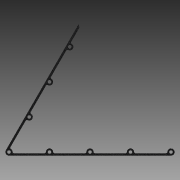
# Autodesk Inventor part: g16-strut1
Saved by Autodesk Inventor 2013 (Build 170138000, 138)
## iProperties
Created: 2013-03-23
Part Number: g16-strut1
Material: Acrylic
Document SubType Name: Modeling
Designer: Beth Scott
Density: 1 g/cm^3
d0: 1.000 ul
d2: 3.000 mm
Strut_Thickness: 2.000 mm
d12: 2.000 mm
d13: 2.000 mm
d14: 2.000 mm
Strut_MateAngle: 135.00 deg
d16: 2.000 mm
d17: 2.000 mm
Strut_Separation: 0.001 mm
d26: 2.000 mm
d27: 2.000 mm
d28: 2.000 mm
ThickLayerThickness: 6.000 mm
d30: 0.00 deg
d1: 1.000 ul
d6: 2.750 mm
d7: 0.00 deg
d8: 3.000 mm
d18: 1.000 ul
d20: 1.000 ul
d22: 0.00 deg
Bolt_HeadDiameter: 6.000 mm
LayerThickness: 2.750 mm
d4: 0.00 deg
Bolt_HoleDiameter: 3.000 mm
d19: 0.00 deg
Bolt_HeadDiameter_1: 6.000 mm
LayerThickness_1: 2.750 mm
Bolt_HoleDiameter_1: 3.000 mm
Pixel_BorderWidth_1: 1.000 mm
Pixel_Stride_1: 33.333 mm
Base_SideWidth: 133.332 mm
Pixel_BorderWidth_2: 1.000 mm
Pixel_Stride_2: 33.333 mm
d24_1: 6.000 mm
CardboardThickness: 1.750 mm
LED_StripWidth: 10.250 mm
LED_Package: 5.000 mm
LED_CapW: 2.500 mm
LED_CapH: 6.000 mm
d32: 16.667 mm
d33: 10.250 mm
LED_SlotWidth: 2.000 mm
d36: 2.000 mm
AlignmentNotchDiameter: 2.000 mm
d52: 2.000 mm
d53: 2.000 mm
LED_CapDist: 8.000 mm
d56: 16.667 mm
d61: 16.667 mm
d62: 28.867 mm
Cardboard_BorderThickness: 2.000 mm
Author: Beth Scott
Autodesk Inventor part; units mm, degrees
(part 1 of 2)
ref_plane "YZ Plane" through (0, 0, 0) normal (1, 0, 0) x (0, 1, 0)
ref_plane "XZ Plane" through (0, 0, 0) normal (0, 1, 0) x (-1, 0, 0)
ref_plane "XY Plane" through (0, 0, 0) normal (0, 0, 1) x (1, 0, 0)
sketch "Triangle Hole Template" plane through (0, 0, 0) normal (0, 0, 1) x (1, 0, 0)
  line L0 (-99.9974, -57.7156) -> (-66.6644, -57.7156) construction
  line L1 (-66.6644, -57.7156) -> (-83.3309, -86.5829) construction
  line L2 (-83.3309, -86.5829) -> (-99.9974, -57.7156) construction
  line L3 (-99.1314, -58.2156) -> (-67.5304, -58.2156) construction
  line L4 (-67.5304, -58.2156) -> (-83.3309, -85.5829) construction
  line L5 (-83.3309, -85.5829) -> (-99.1314, -58.2156) construction
  line L6 (-83.3309, -58.2156) -> (-83.3309, -57.7156) construction
  line L7 (-75.4307, -71.8992) -> (-74.9976, -72.1492) construction
  line L8 (-91.2311, -71.8992) -> (-91.6641, -72.1492) construction
  arc A0 (-68.5696, -60.0156) -> (-69.6089, -58.2156) centre (-69.6089, -59.4156) ccw
  arc A1 (-84.3701, -83.7829) -> (-82.2917, -83.7829) centre (-83.3309, -83.1829) ccw
  arc A2 (-97.0529, -58.2156) -> (-98.0921, -60.0156) centre (-97.0529, -59.4156) ccw
  line L9 (-97.0529, -58.2156) -> (-69.6089, -58.2156)
  line L10 (-68.5696, -60.0156) -> (-82.2917, -83.7829)
  line L11 (-84.3701, -83.7829) -> (-98.0921, -60.0156)
  circle A3 centre (-98.4385, -58.6156) radius 0.4 construction
  line L12 (-98.0921, -58.8156) -> (-98.785, -58.4156) construction
  circle A4 centre (-99.9974, -57.7156) radius 3 construction
  line L13 (-83.3309, -57.7156) -> (-83.3309, -57.2156) construction
  line L14 (-98.0921, -58.8156) -> (-97.3993, -59.2156) construction
  point P0 (-85.6081, -66.0431)
sketch "LED Slot Spacer" plane through (0, 0, 0) normal (0, 0, 1) x (1, 0, 0)
  line L0 (134.5658, -38.3134) -> (132.5658, -38.3134) construction
  point P0 (133.5658, -38.3134)
  point P1 (133.5658, -38.3134)
  dimension "d36" = 2
  measures "d36" distance of L0.start L0.end
sketch "LED Slot" plane through (0, 0, 0) normal (0, 0, 1) x (1, 0, 0)
  line L0 (126.9917, -69.5033) -> (126.9917, -59.2533)
  line L1 (128.9917, -69.5033) -> (128.9917, -59.2533)
  arc A0 (126.9917, -69.5033) -> (128.9917, -69.5033) centre (127.9917, -69.5033) ccw
  arc A1 (128.9917, -59.2533) -> (126.9917, -59.2533) centre (127.9917, -59.2533) ccw
  point P0 (127.9917, -64.3783)
  dimension "d33" = 10.25
  dimension "LED_SlotWidth" = 2
  measures "d33" distance of L0.start L0.end
  measures "LED_SlotWidth" distance of L0.start L1.start
sketch "LED Keepout Regions" plane through (0, 0, 0) normal (0, 0, 1) x (1, 0, 0)
  line L0 (120.8464, -124.1742) -> (104.1799, -124.1742) construction
  line L1 (104.1799, -124.1742) -> (104.1799, -113.9242) construction
  line L2 (104.1799, -113.9242) -> (120.8464, -113.9242) construction
  line L3 (120.8464, -113.9242) -> (120.8464, -124.1742) construction
  line L4 (115.0132, -121.5492) -> (110.0132, -121.5492) construction
  line L5 (110.0132, -121.5492) -> (110.0132, -116.5492) construction
  line L6 (110.0132, -116.5492) -> (115.0132, -116.5492) construction
  line L7 (115.0132, -116.5492) -> (115.0132, -121.5492) construction
  line L8 (112.5132, -124.1742) -> (112.5132, -113.9242) construction
  line L9 (120.8464, -119.0492) -> (104.1799, -119.0492) construction
  line L10 (109.5132, -122.0492) -> (107.0132, -122.0492) construction
  line L11 (107.0132, -122.0492) -> (107.0132, -116.0492) construction
  line L12 (107.0132, -116.0492) -> (109.5132, -116.0492) construction
  line L13 (109.5132, -116.0492) -> (109.5132, -122.0492) construction
  line L14 (117.0132, -113.9242) -> (117.0132, -124.1742) construction
  line L15 (105.0132, -113.9242) -> (105.0132, -124.1742) construction
  point P0 (111.5921, -119.1808)
  point P1 (115.0132, -119.0492)
  point P2 (112.5132, -121.5492)
  point P3 (109.5132, -119.0492)
  dimension "LED_StripWidth" = 10.25
  dimension "LED_Package" = 5
  dimension "LED_CapW" = 2.5
  dimension "LED_CapH" = 6
  dimension "d32" = 16.6665
  dimension "d52" = 2
  dimension "d53" = 2
  dimension "LED_CapDist" = 8
  measures "LED_StripWidth" distance of L2.end L0.start
  measures "LED_Package" distance of L4.start L4.end
  measures "LED_CapW" distance of L10.start L10.end
  measures "LED_CapH" distance of L10.end L11.end
  measures "d32" distance of L1.end L2.end
  measures "d52" distance between parallel lines of L11 L15
  measures "d53" distance between parallel lines of L14 L7
  measures "LED_CapDist" distance between parallel lines of L7 L11
sketch "Triangle Hole Template_1" plane through (0, 0, 0) normal (0, 0, 1) x (1, 0, 0)
  line L0 (-99.9974, -57.7156) -> (-66.6644, -57.7156) construction
  line L1 (-66.6644, -57.7156) -> (-83.3309, -86.5829) construction
  line L2 (-83.3309, -86.5829) -> (-99.9974, -57.7156) construction
  line L3 (-99.1314, -58.2156) -> (-67.5304, -58.2156) construction
  line L4 (-83.3309, -57.7156) -> (-83.3309, -57.2156) construction
  line L5 (-98.0921, -58.8156) -> (-97.3993, -59.2156) construction
  line L6 (-67.5304, -58.2156) -> (-83.3309, -85.5829) construction
  line L7 (-83.3309, -85.5829) -> (-99.1314, -58.2156) construction
  line L8 (-83.3309, -58.2156) -> (-83.3309, -57.7156) construction
  line L9 (-75.4307, -71.8992) -> (-74.9976, -72.1492) construction
  line L10 (-91.2311, -71.8992) -> (-91.6641, -72.1492) construction
  arc A0 (-68.5696, -60.0156) -> (-69.6089, -58.2156) centre (-69.6089, -59.4156) ccw
  arc A1 (-84.3701, -83.7829) -> (-82.2917, -83.7829) centre (-83.3309, -83.1829) ccw
  arc A2 (-97.0529, -58.2156) -> (-98.0921, -60.0156) centre (-97.0529, -59.4156) ccw
  line L11 (-97.0529, -58.2156) -> (-69.6089, -58.2156)
  line L12 (-68.5696, -60.0156) -> (-82.2917, -83.7829)
  line L13 (-84.3701, -83.7829) -> (-98.0921, -60.0156)
  circle A3 centre (-98.4385, -58.6156) radius 0.4 construction
  line L14 (-98.0921, -58.8156) -> (-98.785, -58.4156) construction
  circle A4 centre (-99.9974, -57.7156) radius 3 construction
  point P0 (-85.6081, -66.0431)
sketch "Triangle Hole Template x16" plane through (0, 0, 0) normal (0, 0, 1) x (1, 0, 0)
  line L0 (-99.9974, -57.7156) -> (-66.6644, -57.7156) construction
  line L1 (-66.6644, -57.7156) -> (-83.3309, -86.5829) construction
  line L2 (-83.3309, -86.5829) -> (-99.9974, -57.7156) construction
  line L3 (-99.1314, -58.2156) -> (-67.5304, -58.2156) construction
  line L4 (-67.5304, -58.2156) -> (-83.3309, -85.5829) construction
  line L5 (-83.3309, -85.5829) -> (-99.1314, -58.2156) construction
  line L6 (-83.3309, -58.2156) -> (-83.3309, -57.7156) construction
  line L7 (-75.4307, -71.8992) -> (-74.9976, -72.1492) construction
  line L8 (-91.2311, -71.8992) -> (-91.6641, -72.1492) construction
  arc A0 (-68.5696, -60.0156) -> (-69.6089, -58.2156) centre (-69.6089, -59.4156) ccw
  arc A1 (-84.3701, -83.7829) -> (-82.2917, -83.7829) centre (-83.3309, -83.1829) ccw
  arc A2 (-97.0529, -58.2156) -> (-98.0921, -60.0156) centre (-97.0529, -59.4156) ccw
  line L9 (-97.0529, -58.2156) -> (-69.6089, -58.2156)
  line L10 (-68.5696, -60.0156) -> (-82.2917, -83.7829)
  line L11 (-84.3701, -83.7829) -> (-98.0921, -60.0156)
  circle A3 centre (-98.4385, -58.6156) radius 0.4 construction
  line L12 (-98.0921, -58.8156) -> (-98.785, -58.4156) construction
  circle A4 centre (-99.9974, -57.7156) radius 3 construction
  line L13 (-83.3309, -57.7156) -> (-83.3309, -57.2156) construction
  line L14 (-98.0921, -58.8156) -> (-97.3993, -59.2156) construction
  line L15 (-83.3309, -86.5829) -> (-49.9979, -86.5829) construction
  line L16 (-49.9979, -86.5829) -> (-66.6644, -115.4501) construction
  line L17 (-66.6644, -115.4501) -> (-83.3309, -86.5829) construction
  line L18 (-82.4649, -87.0829) -> (-50.8639, -87.0829) construction
  line L19 (-50.8639, -87.0829) -> (-66.6644, -114.4501) construction
  line L20 (-66.6644, -114.4501) -> (-82.4649, -87.0829) construction
  line L21 (-66.6644, -87.0829) -> (-66.6644, -86.5829) construction
  line L22 (-58.7642, -100.7665) -> (-58.3311, -101.0165) construction
  line L23 (-74.5646, -100.7665) -> (-74.9976, -101.0165) construction
  arc A5 (-51.9031, -88.8829) -> (-52.9424, -87.0829) centre (-52.9424, -88.2829) ccw
  arc A6 (-67.7036, -112.6501) -> (-65.6252, -112.6501) centre (-66.6644, -112.0501) ccw
  arc A7 (-80.3864, -87.0829) -> (-81.4256, -88.8829) centre (-80.3864, -88.2829) ccw
  line L24 (-80.3864, -87.0829) -> (-52.9424, -87.0829)
  line L25 (-51.9031, -88.8829) -> (-65.6252, -112.6501)
  line L26 (-67.7036, -112.6501) -> (-81.4256, -88.8829)
  circle A8 centre (-81.772, -87.4829) radius 0.4 construction
  line L27 (-81.4256, -87.6829) -> (-82.1185, -87.2829) construction
  circle A9 centre (-83.3309, -86.5829) radius 3 construction
  line L28 (-66.6644, -86.5829) -> (-66.6644, -86.0829) construction
  line L29 (-81.4256, -87.6829) -> (-80.7328, -88.0829) construction
  line L30 (-66.6676, -57.7533) -> (-33.3346, -57.7533) construction
  line L31 (-33.3346, -57.7533) -> (-50.0011, -86.6205) construction
  line L32 (-50.0011, -86.6205) -> (-66.6676, -57.7533) construction
  line L33 (-65.8016, -58.2533) -> (-34.2006, -58.2533) construction
  line L34 (-34.2006, -58.2533) -> (-50.0011, -85.6205) construction
  line L35 (-50.0011, -85.6205) -> (-65.8016, -58.2533) construction
  line L36 (-50.0011, -58.2533) -> (-50.0011, -57.7533) construction
  line L37 (-42.1009, -71.9369) -> (-41.6679, -72.1869) construction
  line L38 (-57.9013, -71.9369) -> (-58.3344, -72.1869) construction
  arc A10 (-35.2399, -60.0533) -> (-36.2791, -58.2533) centre (-36.2791, -59.4533) ccw
  arc A11 (-51.0403, -83.8205) -> (-48.9619, -83.8205) centre (-50.0011, -83.2205) ccw
  arc A12 (-63.7231, -58.2533) -> (-64.7624, -60.0533) centre (-63.7231, -59.4533) ccw
  line L39 (-63.7231, -58.2533) -> (-36.2791, -58.2533)
  line L40 (-35.2399, -60.0533) -> (-48.9619, -83.8205)
  line L41 (-51.0403, -83.8205) -> (-64.7624, -60.0533)
  circle A13 centre (-65.1088, -58.6533) radius 0.4 construction
  line L42 (-64.7624, -58.8533) -> (-65.4552, -58.4533) construction
  circle A14 centre (-66.6676, -57.7533) radius 3 construction
  line L43 (-50.0011, -57.7533) -> (-50.0011, -57.2533) construction
  line L44 (-64.7624, -58.8533) -> (-64.0695, -59.2533) construction
  line L45 (-50.0011, -86.6205) -> (-83.3341, -86.6205) construction
  line L46 (-83.3341, -86.6205) -> (-66.6676, -57.7533) construction
  line L47 (-66.6676, -57.7533) -> (-50.0011, -86.6205) construction
  line L48 (-50.8671, -86.1205) -> (-82.4681, -86.1205) construction
  line L49 (-82.4681, -86.1205) -> (-66.6676, -58.7533) construction
  line L50 (-66.6676, -58.7533) -> (-50.8671, -86.1205) construction
  line L51 (-66.6676, -86.1205) -> (-66.6676, -86.6205) construction
  line L52 (-74.5678, -72.4369) -> (-75.0009, -72.1869) construction
  line L53 (-58.7674, -72.4369) -> (-58.3344, -72.1869) construction
  arc A15 (-81.4289, -84.3205) -> (-80.3896, -86.1205) centre (-80.3896, -84.9205) ccw
  arc A16 (-65.6284, -60.5533) -> (-67.7068, -60.5533) centre (-66.6676, -61.1533) ccw
  arc A17 (-52.9456, -86.1205) -> (-51.9064, -84.3205) centre (-52.9456, -84.9205) ccw
  line L54 (-52.9456, -86.1205) -> (-80.3896, -86.1205)
  line L55 (-81.4289, -84.3205) -> (-67.7068, -60.5533)
  line L56 (-65.6284, -60.5533) -> (-51.9064, -84.3205)
  circle A18 centre (-51.56, -85.7205) radius 0.4 construction
  line L57 (-51.9064, -85.5205) -> (-51.2135, -85.9205) construction
  circle A19 centre (-50.0011, -86.6205) radius 3 construction
  line L58 (-66.6676, -86.6205) -> (-66.6676, -87.1205) construction
  line L59 (-51.9064, -85.5205) -> (-52.5992, -85.1205) construction
  line L60 (-33.3346, -57.7533) -> (-66.6676, -57.7533) construction
  line L61 (-66.6676, -57.7533) -> (-50.0011, -28.886) construction
  line L62 (-50.0011, -28.886) -> (-33.3346, -57.7533) construction
  line L63 (-34.2006, -57.2533) -> (-65.8016, -57.2533) construction
  line L64 (-65.8016, -57.2533) -> (-50.0011, -29.886) construction
  line L65 (-50.0011, -29.886) -> (-34.2006, -57.2533) construction
  line L66 (-50.0011, -57.2533) -> (-50.0011, -57.7533) construction
  line L67 (-57.9013, -43.5697) -> (-58.3344, -43.3197) construction
  line L68 (-42.1009, -43.5697) -> (-41.6679, -43.3197) construction
  arc A20 (-64.7624, -55.4533) -> (-63.7231, -57.2533) centre (-63.7231, -56.0533) ccw
  arc A21 (-48.9619, -31.686) -> (-51.0403, -31.686) centre (-50.0011, -32.286) ccw
  arc A22 (-36.2791, -57.2533) -> (-35.2399, -55.4533) centre (-36.2791, -56.0533) ccw
  line L69 (-36.2791, -57.2533) -> (-63.7231, -57.2533)
  line L70 (-64.7624, -55.4533) -> (-51.0403, -31.686)
  line L71 (-48.9619, -31.686) -> (-35.2399, -55.4533)
  circle A23 centre (-34.8935, -56.8533) radius 0.4 construction
  line L72 (-35.2399, -56.6533) -> (-34.547, -57.0533) construction
  circle A24 centre (-33.3346, -57.7533) radius 3 construction
  line L73 (-50.0011, -57.7533) -> (-50.0011, -58.2533) construction
  line L74 (-35.2399, -56.6533) -> (-35.9327, -56.2533) construction
  line L75 (-66.6676, -57.7156) -> (-100.0006, -57.7156) construction
  line L76 (-100.0006, -57.7156) -> (-83.3341, -28.8484) construction
  line L77 (-83.3341, -28.8484) -> (-66.6676, -57.7156) construction
  line L78 (-67.5336, -57.2156) -> (-99.1346, -57.2156) construction
  line L79 (-99.1346, -57.2156) -> (-83.3341, -29.8484) construction
  line L80 (-83.3341, -29.8484) -> (-67.5336, -57.2156) construction
  line L81 (-83.3341, -57.2156) -> (-83.3341, -57.7156) construction
  line L82 (-91.2343, -43.532) -> (-91.6674, -43.282) construction
  line L83 (-75.4339, -43.532) -> (-75.0009, -43.282) construction
  arc A25 (-98.0954, -55.4156) -> (-97.0561, -57.2156) centre (-97.0561, -56.0156) ccw
  arc A26 (-82.2949, -31.6484) -> (-84.3733, -31.6484) centre (-83.3341, -32.2484) ccw
  arc A27 (-69.6121, -57.2156) -> (-68.5729, -55.4156) centre (-69.6121, -56.0156) ccw
  line L84 (-69.6121, -57.2156) -> (-97.0561, -57.2156)
  line L85 (-98.0954, -55.4156) -> (-84.3733, -31.6484)
  line L86 (-82.2949, -31.6484) -> (-68.5729, -55.4156)
  circle A28 centre (-68.2265, -56.8156) radius 0.4 construction
  line L87 (-68.5729, -56.6156) -> (-67.88, -57.0156) construction
  circle A29 centre (-66.6676, -57.7156) radius 3 construction
  line L88 (-83.3341, -57.7156) -> (-83.3341, -58.2156) construction
  line L89 (-68.5729, -56.6156) -> (-69.2657, -56.2156) construction
  line L90 (-83.3186, -28.8752) -> (-116.6516, -28.8752) construction
  line L91 (-116.6516, -28.8752) -> (-99.9851, -0.008) construction
  line L92 (-99.9851, -0.008) -> (-83.3186, -28.8752) construction
  line L93 (-84.1846, -28.3752) -> (-115.7856, -28.3752) construction
  line L94 (-115.7856, -28.3752) -> (-99.9851, -1.008) construction
  line L95 (-99.9851, -1.008) -> (-84.1846, -28.3752) construction
  line L96 (-99.9851, -28.3752) -> (-99.9851, -28.8752) construction
  line L97 (-107.8853, -14.6916) -> (-108.3184, -14.4416) construction
  line L98 (-92.0849, -14.6916) -> (-91.6519, -14.4416) construction
  arc A30 (-114.7464, -26.5752) -> (-113.7071, -28.3752) centre (-113.7071, -27.1752) ccw
  arc A31 (-98.9459, -2.808) -> (-101.0243, -2.808) centre (-99.9851, -3.408) ccw
  arc A32 (-86.2631, -28.3752) -> (-85.2239, -26.5752) centre (-86.2631, -27.1752) ccw
  line L99 (-86.2631, -28.3752) -> (-113.7071, -28.3752)
  line L100 (-114.7464, -26.5752) -> (-101.0243, -2.808)
  line L101 (-98.9459, -2.808) -> (-85.2239, -26.5752)
  circle A33 centre (-84.8775, -27.9752) radius 0.4 construction
  line L102 (-85.2239, -27.7752) -> (-84.531, -28.1752) construction
  circle A34 centre (-83.3186, -28.8752) radius 3 construction
  line L103 (-99.9851, -28.8752) -> (-99.9851, -29.3752) construction
  line L104 (-85.2239, -27.7752) -> (-85.9167, -27.3752) construction
  line L105 (-50.0011, -28.8484) -> (-83.3341, -28.8484) construction
  line L106 (-83.3341, -28.8484) -> (-66.6676, 0.0188) construction
  line L107 (-66.6676, 0.0188) -> (-50.0011, -28.8484) construction
  line L108 (-50.8671, -28.3484) -> (-82.4681, -28.3484) construction
  line L109 (-82.4681, -28.3484) -> (-66.6676, -0.9812) construction
  line L110 (-66.6676, -0.9812) -> (-50.8671, -28.3484) construction
  line L111 (-66.6676, -28.3484) -> (-66.6676, -28.8484) construction
  line L112 (-74.5678, -14.6648) -> (-75.0009, -14.4148) construction
  line L113 (-58.7674, -14.6648) -> (-58.3344, -14.4148) construction
  arc A35 (-81.4289, -26.5484) -> (-80.3896, -28.3484) centre (-80.3896, -27.1484) ccw
  arc A36 (-65.6284, -2.7812) -> (-67.7068, -2.7812) centre (-66.6676, -3.3812) ccw
  arc A37 (-52.9456, -28.3484) -> (-51.9064, -26.5484) centre (-52.9456, -27.1484) ccw
  line L114 (-52.9456, -28.3484) -> (-80.3896, -28.3484)
  line L115 (-81.4289, -26.5484) -> (-67.7068, -2.7812)
  line L116 (-65.6284, -2.7812) -> (-51.9064, -26.5484)
  circle A38 centre (-51.56, -27.9484) radius 0.4 construction
  line L117 (-51.9064, -27.7484) -> (-51.2135, -28.1484) construction
  circle A39 centre (-50.0011, -28.8484) radius 3 construction
  line L118 (-66.6676, -28.8484) -> (-66.6676, -29.3484) construction
  line L119 (-51.9064, -27.7484) -> (-52.5992, -27.3484) construction
  line L120 (-16.6681, -28.8484) -> (-50.0011, -28.8484) construction
  line L121 (-50.0011, -28.8484) -> (-33.3346, 0.0188) construction
  line L122 (-33.3346, 0.0188) -> (-16.6681, -28.8484) construction
  line L123 (-17.5341, -28.3484) -> (-49.1351, -28.3484) construction
  line L124 (-49.1351, -28.3484) -> (-33.3346, -0.9812) construction
  line L125 (-33.3346, -0.9812) -> (-17.5341, -28.3484) construction
  line L126 (-33.3346, -28.3484) -> (-33.3346, -28.8484) construction
  line L127 (-41.2348, -14.6648) -> (-41.6679, -14.4148) construction
  line L128 (-25.4344, -14.6648) -> (-25.0014, -14.4148) construction
  arc A40 (-48.0959, -26.5484) -> (-47.0566, -28.3484) centre (-47.0566, -27.1484) ccw
  arc A41 (-32.2954, -2.7812) -> (-34.3738, -2.7812) centre (-33.3346, -3.3812) ccw
  arc A42 (-19.6126, -28.3484) -> (-18.5734, -26.5484) centre (-19.6126, -27.1484) ccw
  line L129 (-19.6126, -28.3484) -> (-47.0566, -28.3484)
  line L130 (-48.0959, -26.5484) -> (-34.3738, -2.7812)
  line L131 (-32.2954, -2.7812) -> (-18.5734, -26.5484)
  circle A43 centre (-18.227, -27.9484) radius 0.4 construction
  line L132 (-18.5734, -27.7484) -> (-17.8805, -28.1484) construction
  circle A44 centre (-16.6681, -28.8484) radius 3 construction
  line L133 (-33.3346, -28.8484) -> (-33.3346, -29.3484) construction
  line L134 (-18.5734, -27.7484) -> (-19.2662, -27.3484) construction
  line L135 (-49.9979, -28.8484) -> (-16.6649, -28.8484) construction
  line L136 (-16.6649, -28.8484) -> (-33.3314, -57.7156) construction
  line L137 (-33.3314, -57.7156) -> (-49.9979, -28.8484) construction
  line L138 (-49.1319, -29.3484) -> (-17.5309, -29.3484) construction
  line L139 (-17.5309, -29.3484) -> (-33.3314, -56.7156) construction
  line L140 (-33.3314, -56.7156) -> (-49.1319, -29.3484) construction
  line L141 (-33.3314, -29.3484) -> (-33.3314, -28.8484) construction
  line L142 (-25.4312, -43.032) -> (-24.9981, -43.282) construction
  line L143 (-41.2316, -43.032) -> (-41.6646, -43.282) construction
  arc A45 (-18.5701, -31.1484) -> (-19.6094, -29.3484) centre (-19.6094, -30.5484) ccw
  arc A46 (-34.3706, -54.9156) -> (-32.2922, -54.9156) centre (-33.3314, -54.3156) ccw
  arc A47 (-47.0534, -29.3484) -> (-48.0926, -31.1484) centre (-47.0534, -30.5484) ccw
  line L144 (-47.0534, -29.3484) -> (-19.6094, -29.3484)
  line L145 (-18.5701, -31.1484) -> (-32.2922, -54.9156)
  line L146 (-34.3706, -54.9156) -> (-48.0926, -31.1484)
  circle A48 centre (-48.439, -29.7484) radius 0.4 construction
  line L147 (-48.0926, -29.9484) -> (-48.7855, -29.5484) construction
  circle A49 centre (-49.9979, -28.8484) radius 3 construction
  line L148 (-33.3314, -28.8484) -> (-33.3314, -28.3484) construction
  line L149 (-48.0926, -29.9484) -> (-47.3998, -30.3484) construction
  line L150 (-66.6676, 0.0188) -> (-33.3346, 0.0188) construction
  line L151 (-33.3346, 0.0188) -> (-50.0011, -28.8484) construction
  line L152 (-50.0011, -28.8484) -> (-66.6676, 0.0188) construction
  line L153 (-65.8016, -0.4812) -> (-34.2006, -0.4812) construction
  line L154 (-34.2006, -0.4812) -> (-50.0011, -27.8484) construction
  line L155 (-50.0011, -27.8484) -> (-65.8016, -0.4812) construction
  line L156 (-50.0011, -0.4812) -> (-50.0011, 0.0188) construction
  line L157 (-42.1009, -14.1648) -> (-41.6679, -14.4148) construction
  line L158 (-57.9013, -14.1648) -> (-58.3344, -14.4148) construction
  arc A50 (-35.2399, -2.2812) -> (-36.2791, -0.4812) centre (-36.2791, -1.6812) ccw
  arc A51 (-51.0403, -26.0484) -> (-48.9619, -26.0484) centre (-50.0011, -25.4484) ccw
  arc A52 (-63.7231, -0.4812) -> (-64.7624, -2.2812) centre (-63.7231, -1.6812) ccw
  line L159 (-63.7231, -0.4812) -> (-36.2791, -0.4812)
  line L160 (-35.2399, -2.2812) -> (-48.9619, -26.0484)
  line L161 (-51.0403, -26.0484) -> (-64.7624, -2.2812)
  circle A53 centre (-65.1088, -0.8812) radius 0.4 construction
  line L162 (-64.7624, -1.0812) -> (-65.4552, -0.6812) construction
  circle A54 centre (-66.6676, 0.0188) radius 3 construction
  line L163 (-50.0011, 0.0188) -> (-50.0011, 0.5188) construction
  line L164 (-64.7624, -1.0812) -> (-64.0695, -1.4812) construction
  line L165 (-33.3314, 0.0188) -> (0.0016, 0.0188) construction
  line L166 (0.0016, 0.0188) -> (-16.6649, -28.8484) construction
  line L167 (-16.6649, -28.8484) -> (-33.3314, 0.0188) construction
  line L168 (-32.4654, -0.4812) -> (-0.8644, -0.4812) construction
  line L169 (-0.8644, -0.4812) -> (-16.6649, -27.8484) construction
  line L170 (-16.6649, -27.8484) -> (-32.4654, -0.4812) construction
  line L171 (-16.6649, -0.4812) -> (-16.6649, 0.0188) construction
  line L172 (-8.7647, -14.1648) -> (-8.3316, -14.4148) construction
  line L173 (-24.5651, -14.1648) -> (-24.9981, -14.4148) construction
  arc A55 (-1.9036, -2.2812) -> (-2.9429, -0.4812) centre (-2.9429, -1.6812) ccw
  arc A56 (-17.7041, -26.0484) -> (-15.6257, -26.0484) centre (-16.6649, -25.4484) ccw
  arc A57 (-30.3869, -0.4812) -> (-31.4261, -2.2812) centre (-30.3869, -1.6812) ccw
  line L174 (-30.3869, -0.4812) -> (-2.9429, -0.4812)
  line L175 (-1.9036, -2.2812) -> (-15.6257, -26.0484)
  line L176 (-17.7041, -26.0484) -> (-31.4261, -2.2812)
  circle A58 centre (-31.7725, -0.8812) radius 0.4 construction
  line L177 (-31.4261, -1.0812) -> (-32.119, -0.6812) construction
  circle A59 centre (-33.3314, 0.0188) radius 3 construction
  line L178 (-16.6649, 0.0188) -> (-16.6649, 0.5188) construction
  line L179 (-31.4261, -1.0812) -> (-30.7333, -1.4812) construction
  line L180 (-83.317, -28.8188) -> (-49.984, -28.8188) construction
  line L181 (-49.984, -28.8188) -> (-66.6505, -57.686) construction
  line L182 (-66.6505, -57.686) -> (-83.317, -28.8188) construction
  line L183 (-82.451, -29.3188) -> (-50.85, -29.3188) construction
  line L184 (-50.85, -29.3188) -> (-66.6505, -56.686) construction
  line L185 (-66.6505, -56.686) -> (-82.451, -29.3188) construction
  line L186 (-66.6505, -29.3188) -> (-66.6505, -28.8188) construction
  line L187 (-58.7503, -43.0024) -> (-58.3173, -43.2524) construction
  line L188 (-74.5507, -43.0024) -> (-74.9838, -43.2524) construction
  arc A60 (-51.8893, -31.1188) -> (-52.9285, -29.3188) centre (-52.9285, -30.5188) ccw
  arc A61 (-67.6897, -54.886) -> (-65.6113, -54.886) centre (-66.6505, -54.286) ccw
  arc A62 (-80.3725, -29.3188) -> (-81.4117, -31.1188) centre (-80.3725, -30.5188) ccw
  line L189 (-80.3725, -29.3188) -> (-52.9285, -29.3188)
  line L190 (-51.8893, -31.1188) -> (-65.6113, -54.886)
  line L191 (-67.6897, -54.886) -> (-81.4117, -31.1188)
  circle A63 centre (-81.7582, -29.7188) radius 0.4 construction
  line L192 (-81.4117, -29.9188) -> (-82.1046, -29.5188) construction
  circle A64 centre (-83.317, -28.8188) radius 3 construction
  line L193 (-66.6505, -28.8188) -> (-66.6505, -28.3188) construction
  line L194 (-81.4117, -29.9188) -> (-80.7189, -30.3188) construction
  line L195 (-99.9974, 0.0188) -> (-66.6644, 0.0188) construction
  line L196 (-66.6644, 0.0188) -> (-83.3309, -28.8484) construction
  line L197 (-83.3309, -28.8484) -> (-99.9974, 0.0188) construction
  line L198 (-99.1314, -0.4812) -> (-67.5304, -0.4812) construction
  line L199 (-67.5304, -0.4812) -> (-83.3309, -27.8484) construction
  line L200 (-83.3309, -27.8484) -> (-99.1314, -0.4812) construction
  line L201 (-83.3309, -0.4812) -> (-83.3309, 0.0188) construction
  line L202 (-75.4307, -14.1648) -> (-74.9976, -14.4148) construction
  line L203 (-91.2311, -14.1648) -> (-91.6641, -14.4148) construction
  arc A65 (-68.5696, -2.2812) -> (-69.6089, -0.4812) centre (-69.6089, -1.6812) ccw
  arc A66 (-84.3701, -26.0484) -> (-82.2917, -26.0484) centre (-83.3309, -25.4484) ccw
  arc A67 (-97.0529, -0.4812) -> (-98.0921, -2.2812) centre (-97.0529, -1.6812) ccw
  line L204 (-97.0529, -0.4812) -> (-69.6089, -0.4812)
  line L205 (-68.5696, -2.2812) -> (-82.2917, -26.0484)
  line L206 (-84.3701, -26.0484) -> (-98.0921, -2.2812)
  circle A68 centre (-98.4385, -0.8812) radius 0.4 construction
  line L207 (-98.0921, -1.0812) -> (-98.785, -0.6812) construction
  circle A69 centre (-99.9974, 0.0188) radius 3 construction
  line L208 (-83.3309, 0.0188) -> (-83.3309, 0.5188) construction
  line L209 (-98.0921, -1.0812) -> (-97.3993, -1.4812) construction
  line L210 (-133.3304, -0.008) -> (-99.9974, -0.008) construction
  line L211 (-99.9974, -0.008) -> (-116.6639, -28.8752) construction
  line L212 (-116.6639, -28.8752) -> (-133.3304, -0.008) construction
  line L213 (-132.4644, -0.508) -> (-100.8634, -0.508) construction
  line L214 (-100.8634, -0.508) -> (-116.6639, -27.8752) construction
  line L215 (-116.6639, -27.8752) -> (-132.4644, -0.508) construction
  line L216 (-116.6639, -0.508) -> (-116.6639, -0.008) construction
  line L217 (-108.7637, -14.1916) -> (-108.3306, -14.4416) construction
  line L218 (-124.5641, -14.1916) -> (-124.9971, -14.4416) construction
  arc A70 (-101.9026, -2.308) -> (-102.9419, -0.508) centre (-102.9419, -1.708) ccw
  arc A71 (-117.7031, -26.0752) -> (-115.6247, -26.0752) centre (-116.6639, -25.4752) ccw
  arc A72 (-130.3859, -0.508) -> (-131.4251, -2.308) centre (-130.3859, -1.708) ccw
  line L219 (-130.3859, -0.508) -> (-102.9419, -0.508)
  line L220 (-101.9026, -2.308) -> (-115.6247, -26.0752)
  line L221 (-117.7031, -26.0752) -> (-131.4251, -2.308)
  circle A73 centre (-131.7715, -0.908) radius 0.4 construction
  line L222 (-131.4251, -1.108) -> (-132.118, -0.708) construction
  circle A74 centre (-133.3304, -0.008) radius 3 construction
  line L223 (-116.6639, -0.008) -> (-116.6639, 0.492) construction
  line L224 (-131.4251, -1.108) -> (-130.7323, -1.508) construction
  line L225 (-116.6671, -28.8484) -> (-83.3341, -28.8484) construction
  line L226 (-83.3341, -28.8484) -> (-100.0006, -57.7156) construction
  line L227 (-100.0006, -57.7156) -> (-116.6671, -28.8484) construction
  line L228 (-115.8011, -29.3484) -> (-84.2001, -29.3484) construction
  line L229 (-84.2001, -29.3484) -> (-100.0006, -56.7156) construction
  line L230 (-100.0006, -56.7156) -> (-115.8011, -29.3484) construction
  line L231 (-100.0006, -29.3484) -> (-100.0006, -28.8484) construction
  line L232 (-92.1004, -43.032) -> (-91.6674, -43.282) construction
  line L233 (-107.9008, -43.032) -> (-108.3339, -43.282) construction
  arc A75 (-85.2394, -31.1484) -> (-86.2786, -29.3484) centre (-86.2786, -30.5484) ccw
  arc A76 (-101.0398, -54.9156) -> (-98.9614, -54.9156) centre (-100.0006, -54.3156) ccw
  arc A77 (-113.7226, -29.3484) -> (-114.7619, -31.1484) centre (-113.7226, -30.5484) ccw
  line L234 (-113.7226, -29.3484) -> (-86.2786, -29.3484)
  line L235 (-85.2394, -31.1484) -> (-98.9614, -54.9156)
  line L236 (-101.0398, -54.9156) -> (-114.7619, -31.1484)
  circle A78 centre (-115.1083, -29.7484) radius 0.4 construction
  line L237 (-114.7619, -29.9484) -> (-115.4547, -29.5484) construction
  circle A79 centre (-116.6671, -28.8484) radius 3 construction
  line L238 (-100.0006, -28.8484) -> (-100.0006, -28.3484) construction
  line L239 (-114.7619, -29.9484) -> (-114.069, -30.3484) construction
  point P0 (-67.2349, -38.1612)
sketch "LED Keepout x16" plane through (0, 0, 0) normal (0, 0, 1) x (1, 0, 0)
  line L0 (133.3347, -3) -> (0.0027, -3) construction
  line L1 (116.6682, -31.8672) -> (16.6692, -31.8672) construction
  line L2 (83.3352, -89.6017) -> (50.0022, -89.6017) construction
  line L3 (116.6682, -31.8672) -> (116.6682, -3) construction
  line L4 (100.0017, -60.7344) -> (33.3357, -60.7344) construction
  line L5 (100.0017, -60.7344) -> (100.0017, -31.8672) construction
  line L6 (83.3352, -89.6017) -> (83.3352, -60.7344) construction
  line L7 (66.6687, -118.4689) -> (66.6687, -89.6017) construction
  line L8 (50.0022, -89.6017) -> (50.0022, -3) construction
  line L9 (16.6692, -31.8672) -> (16.6692, -3) construction
  line L10 (33.3357, -60.7344) -> (33.3357, -3) construction
  line L11 (66.6687, -89.6017) -> (66.6687, -3) construction
  line L12 (83.3352, -60.7344) -> (83.3352, -3) construction
  line L13 (100.0017, -31.8672) -> (100.0017, -3) construction
  line L14 (125.0015, -22.5586) -> (108.335, -22.5586) construction
  line L15 (108.335, -22.5586) -> (108.335, -12.3086) construction
  line L16 (108.335, -12.3086) -> (125.0015, -12.3086) construction
  line L17 (125.0015, -12.3086) -> (125.0015, -22.5586) construction
  line L18 (119.1682, -19.9336) -> (114.1682, -19.9336) construction
  line L19 (114.1682, -19.9336) -> (114.1682, -14.9336) construction
  line L20 (114.1682, -14.9336) -> (119.1682, -14.9336) construction
  line L21 (119.1682, -14.9336) -> (119.1682, -19.9336) construction
  line L22 (116.6682, -22.5586) -> (116.6682, -12.3086) construction
  line L23 (125.0015, -17.4336) -> (108.335, -17.4336) construction
  line L24 (113.6682, -20.4336) -> (111.1682, -20.4336) construction
  line L25 (111.1682, -20.4336) -> (111.1682, -14.4336) construction
  line L26 (111.1682, -14.4336) -> (113.6682, -14.4336) construction
  line L27 (113.6682, -14.4336) -> (113.6682, -20.4336) construction
  line L28 (121.1682, -12.3086) -> (121.1682, -22.5586) construction
  line L29 (109.1682, -12.3086) -> (109.1682, -22.5586) construction
  line L30 (108.335, -22.5586) -> (91.6685, -22.5586) construction
  line L31 (91.6685, -22.5586) -> (91.6685, -12.3086) construction
  line L32 (91.6685, -12.3086) -> (108.335, -12.3086) construction
  line L33 (108.335, -12.3086) -> (108.335, -22.5586) construction
  line L34 (102.5017, -19.9336) -> (97.5017, -19.9336) construction
  line L35 (97.5017, -19.9336) -> (97.5017, -14.9336) construction
  line L36 (97.5017, -14.9336) -> (102.5017, -14.9336) construction
  line L37 (102.5017, -14.9336) -> (102.5017, -19.9336) construction
  line L38 (100.0017, -22.5586) -> (100.0017, -12.3086) construction
  line L39 (108.335, -17.4336) -> (91.6685, -17.4336) construction
  line L40 (97.0017, -20.4336) -> (94.5017, -20.4336) construction
  line L41 (94.5017, -20.4336) -> (94.5017, -14.4336) construction
  line L42 (94.5017, -14.4336) -> (97.0017, -14.4336) construction
  line L43 (97.0017, -14.4336) -> (97.0017, -20.4336) construction
  line L44 (104.5017, -12.3086) -> (104.5017, -22.5586) construction
  line L45 (92.5017, -12.3086) -> (92.5017, -22.5586) construction
  line L46 (91.6685, -22.5586) -> (75.002, -22.5586) construction
  line L47 (75.002, -22.5586) -> (75.002, -12.3086) construction
  line L48 (75.002, -12.3086) -> (91.6685, -12.3086) construction
  line L49 (91.6685, -12.3086) -> (91.6685, -22.5586) construction
  line L50 (85.8352, -19.9336) -> (80.8352, -19.9336) construction
  line L51 (80.8352, -19.9336) -> (80.8352, -14.9336) construction
  line L52 (80.8352, -14.9336) -> (85.8352, -14.9336) construction
  line L53 (85.8352, -14.9336) -> (85.8352, -19.9336) construction
  line L54 (83.3352, -22.5586) -> (83.3352, -12.3086) construction
  line L55 (91.6685, -17.4336) -> (75.002, -17.4336) construction
  line L56 (80.3352, -20.4336) -> (77.8352, -20.4336) construction
  line L57 (77.8352, -20.4336) -> (77.8352, -14.4336) construction
  line L58 (77.8352, -14.4336) -> (80.3352, -14.4336) construction
  line L59 (80.3352, -14.4336) -> (80.3352, -20.4336) construction
  line L60 (87.8352, -12.3086) -> (87.8352, -22.5586) construction
  line L61 (75.8352, -12.3086) -> (75.8352, -22.5586) construction
  line L62 (75.002, -22.5586) -> (58.3355, -22.5586) construction
  line L63 (58.3355, -22.5586) -> (58.3355, -12.3086) construction
  line L64 (58.3355, -12.3086) -> (75.002, -12.3086) construction
  line L65 (75.002, -12.3086) -> (75.002, -22.5586) construction
  line L66 (69.1687, -19.9336) -> (64.1687, -19.9336) construction
  line L67 (64.1687, -19.9336) -> (64.1687, -14.9336) construction
  line L68 (64.1687, -14.9336) -> (69.1687, -14.9336) construction
  line L69 (69.1687, -14.9336) -> (69.1687, -19.9336) construction
  line L70 (66.6687, -22.5586) -> (66.6687, -12.3086) construction
  line L71 (75.002, -17.4336) -> (58.3355, -17.4336) construction
  line L72 (63.6687, -20.4336) -> (61.1687, -20.4336) construction
  line L73 (61.1687, -20.4336) -> (61.1687, -14.4336) construction
  line L74 (61.1687, -14.4336) -> (63.6687, -14.4336) construction
  line L75 (63.6687, -14.4336) -> (63.6687, -20.4336) construction
  line L76 (71.1687, -12.3086) -> (71.1687, -22.5586) construction
  line L77 (59.1687, -12.3086) -> (59.1687, -22.5586) construction
  line L78 (41.669, -22.5586) -> (25.0025, -22.5586) construction
  line L79 (25.0025, -22.5586) -> (25.0025, -12.3086) construction
  line L80 (25.0025, -12.3086) -> (41.669, -12.3086) construction
  line L81 (41.669, -12.3086) -> (41.669, -22.5586) construction
  line L82 (35.8357, -19.9336) -> (30.8357, -19.9336) construction
  line L83 (30.8357, -19.9336) -> (30.8357, -14.9336) construction
  line L84 (30.8357, -14.9336) -> (35.8357, -14.9336) construction
  line L85 (35.8357, -14.9336) -> (35.8357, -19.9336) construction
  line L86 (33.3357, -22.5586) -> (33.3357, -12.3086) construction
  line L87 (41.669, -17.4336) -> (25.0025, -17.4336) construction
  line L88 (30.3357, -20.4336) -> (27.8357, -20.4336) construction
  line L89 (27.8357, -20.4336) -> (27.8357, -14.4336) construction
  line L90 (27.8357, -14.4336) -> (30.3357, -14.4336) construction
  line L91 (30.3357, -14.4336) -> (30.3357, -20.4336) construction
  line L92 (37.8357, -12.3086) -> (37.8357, -22.5586) construction
  line L93 (25.8357, -12.3086) -> (25.8357, -22.5586) construction
  line L94 (58.3355, -22.5586) -> (41.669, -22.5586) construction
  line L95 (41.669, -22.5586) -> (41.669, -12.3086) construction
  line L96 (41.669, -12.3086) -> (58.3355, -12.3086) construction
  line L97 (58.3355, -12.3086) -> (58.3355, -22.5586) construction
  line L98 (52.5022, -19.9336) -> (47.5022, -19.9336) construction
  line L99 (47.5022, -19.9336) -> (47.5022, -14.9336) construction
  line L100 (47.5022, -14.9336) -> (52.5022, -14.9336) construction
  line L101 (52.5022, -14.9336) -> (52.5022, -19.9336) construction
  line L102 (50.0022, -22.5586) -> (50.0022, -12.3086) construction
  line L103 (58.3355, -17.4336) -> (41.669, -17.4336) construction
  line L104 (47.0022, -20.4336) -> (44.5022, -20.4336) construction
  line L105 (44.5022, -20.4336) -> (44.5022, -14.4336) construction
  line L106 (44.5022, -14.4336) -> (47.0022, -14.4336) construction
  line L107 (47.0022, -14.4336) -> (47.0022, -20.4336) construction
  line L108 (54.5022, -12.3086) -> (54.5022, -22.5586) construction
  line L109 (42.5022, -12.3086) -> (42.5022, -22.5586) construction
  line L110 (25.0025, -22.5586) -> (8.336, -22.5586) construction
  line L111 (8.336, -22.5586) -> (8.336, -12.3086) construction
  line L112 (8.336, -12.3086) -> (25.0025, -12.3086) construction
  line L113 (25.0025, -12.3086) -> (25.0025, -22.5586) construction
  line L114 (19.1692, -19.9336) -> (14.1692, -19.9336) construction
  line L115 (14.1692, -19.9336) -> (14.1692, -14.9336) construction
  line L116 (14.1692, -14.9336) -> (19.1692, -14.9336) construction
  line L117 (19.1692, -14.9336) -> (19.1692, -19.9336) construction
  line L118 (16.6692, -22.5586) -> (16.6692, -12.3086) construction
  line L119 (25.0025, -17.4336) -> (8.336, -17.4336) construction
  line L120 (13.6692, -20.4336) -> (11.1692, -20.4336) construction
  line L121 (11.1692, -20.4336) -> (11.1692, -14.4336) construction
  line L122 (11.1692, -14.4336) -> (13.6692, -14.4336) construction
  line L123 (13.6692, -14.4336) -> (13.6692, -20.4336) construction
  line L124 (21.1692, -12.3086) -> (21.1692, -22.5586) construction
  line L125 (9.1692, -12.3086) -> (9.1692, -22.5586) construction
  line L126 (75.002, -80.2931) -> (58.3355, -80.2931) construction
  line L127 (58.3355, -80.2931) -> (58.3355, -70.0431) construction
  line L128 (58.3355, -70.0431) -> (75.002, -70.0431) construction
  line L129 (75.002, -70.0431) -> (75.002, -80.2931) construction
  line L130 (69.1687, -77.6681) -> (64.1687, -77.6681) construction
  line L131 (64.1687, -77.6681) -> (64.1687, -72.6681) construction
  line L132 (64.1687, -72.6681) -> (69.1687, -72.6681) construction
  line L133 (69.1687, -72.6681) -> (69.1687, -77.6681) construction
  line L134 (66.6687, -80.2931) -> (66.6687, -70.0431) construction
  line L135 (75.002, -75.1681) -> (58.3355, -75.1681) construction
  line L136 (63.6687, -78.1681) -> (61.1687, -78.1681) construction
  line L137 (61.1687, -78.1681) -> (61.1687, -72.1681) construction
  line L138 (61.1687, -72.1681) -> (63.6687, -72.1681) construction
  line L139 (63.6687, -72.1681) -> (63.6687, -78.1681) construction
  line L140 (71.1687, -70.0431) -> (71.1687, -80.2931) construction
  line L141 (59.1687, -70.0431) -> (59.1687, -80.2931) construction
  line L142 (58.3355, -80.2931) -> (41.669, -80.2931) construction
  line L143 (41.669, -80.2931) -> (41.669, -70.0431) construction
  line L144 (41.669, -70.0431) -> (58.3355, -70.0431) construction
  line L145 (58.3355, -70.0431) -> (58.3355, -80.2931) construction
  line L146 (52.5022, -77.6681) -> (47.5022, -77.6681) construction
  line L147 (47.5022, -77.6681) -> (47.5022, -72.6681) construction
  line L148 (47.5022, -72.6681) -> (52.5022, -72.6681) construction
  line L149 (52.5022, -72.6681) -> (52.5022, -77.6681) construction
  line L150 (50.0022, -80.2931) -> (50.0022, -70.0431) construction
  line L151 (58.3355, -75.1681) -> (41.669, -75.1681) construction
  line L152 (47.0022, -78.1681) -> (44.5022, -78.1681) construction
  line L153 (44.5022, -78.1681) -> (44.5022, -72.1681) construction
  line L154 (44.5022, -72.1681) -> (47.0022, -72.1681) construction
  line L155 (47.0022, -72.1681) -> (47.0022, -78.1681) construction
  line L156 (54.5022, -70.0431) -> (54.5022, -80.2931) construction
  line L157 (42.5022, -70.0431) -> (42.5022, -80.2931) construction
  line L158 (25.0025, -41.1758) -> (41.669, -41.1758) construction
  line L159 (41.669, -41.1758) -> (41.669, -51.4258) construction
  line L160 (41.669, -51.4258) -> (25.0025, -51.4258) construction
  line L161 (25.0025, -51.4258) -> (25.0025, -41.1758) construction
  line L162 (30.8357, -43.8008) -> (35.8357, -43.8008) construction
  line L163 (35.8357, -43.8008) -> (35.8357, -48.8008) construction
  line L164 (35.8357, -48.8008) -> (30.8357, -48.8008) construction
  line L165 (30.8357, -48.8008) -> (30.8357, -43.8008) construction
  line L166 (33.3357, -41.1758) -> (33.3357, -51.4258) construction
  line L167 (25.0025, -46.3008) -> (41.669, -46.3008) construction
  line L168 (36.3357, -43.3008) -> (38.8357, -43.3008) construction
  line L169 (38.8357, -43.3008) -> (38.8357, -49.3008) construction
  line L170 (38.8357, -49.3008) -> (36.3357, -49.3008) construction
  line L171 (36.3357, -49.3008) -> (36.3357, -43.3008) construction
  line L172 (28.8357, -51.4258) -> (28.8357, -41.1758) construction
  line L173 (40.8357, -51.4258) -> (40.8357, -41.1758) construction
  line L174 (91.6685, -80.2931) -> (75.002, -80.2931) construction
  line L175 (75.002, -80.2931) -> (75.002, -70.0431) construction
  line L176 (75.002, -70.0431) -> (91.6685, -70.0431) construction
  line L177 (91.6685, -70.0431) -> (91.6685, -80.2931) construction
  line L178 (85.8352, -77.6681) -> (80.8352, -77.6681) construction
  line L179 (80.8352, -77.6681) -> (80.8352, -72.6681) construction
  line L180 (80.8352, -72.6681) -> (85.8352, -72.6681) construction
  line L181 (85.8352, -72.6681) -> (85.8352, -77.6681) construction
  line L182 (83.3352, -80.2931) -> (83.3352, -70.0431) construction
  line L183 (91.6685, -75.1681) -> (75.002, -75.1681) construction
  line L184 (80.3352, -78.1681) -> (77.8352, -78.1681) construction
  line L185 (77.8352, -78.1681) -> (77.8352, -72.1681) construction
  line L186 (77.8352, -72.1681) -> (80.3352, -72.1681) construction
  line L187 (80.3352, -72.1681) -> (80.3352, -78.1681) construction
  line L188 (87.8352, -70.0431) -> (87.8352, -80.2931) construction
  line L189 (75.8352, -70.0431) -> (75.8352, -80.2931) construction
  line L190 (58.3355, -41.1758) -> (75.002, -41.1758) construction
  line L191 (75.002, -41.1758) -> (75.002, -51.4258) construction
  line L192 (75.002, -51.4258) -> (58.3355, -51.4258) construction
  line L193 (58.3355, -51.4258) -> (58.3355, -41.1758) construction
  line L194 (64.1687, -43.8008) -> (69.1687, -43.8008) construction
  line L195 (69.1687, -43.8008) -> (69.1687, -48.8008) construction
  line L196 (69.1687, -48.8008) -> (64.1687, -48.8008) construction
  line L197 (64.1687, -48.8008) -> (64.1687, -43.8008) construction
  line L198 (66.6687, -41.1758) -> (66.6687, -51.4258) construction
  line L199 (58.3355, -46.3008) -> (75.002, -46.3008) construction
  line L200 (69.6687, -43.3008) -> (72.1687, -43.3008) construction
  line L201 (72.1687, -43.3008) -> (72.1687, -49.3008) construction
  line L202 (72.1687, -49.3008) -> (69.6687, -49.3008) construction
  line L203 (69.6687, -49.3008) -> (69.6687, -43.3008) construction
  line L204 (62.1687, -51.4258) -> (62.1687, -41.1758) construction
  line L205 (74.1687, -51.4258) -> (74.1687, -41.1758) construction
  line L206 (75.002, -41.1758) -> (91.6685, -41.1758) construction
  line L207 (91.6685, -41.1758) -> (91.6685, -51.4258) construction
  line L208 (91.6685, -51.4258) -> (75.002, -51.4258) construction
  line L209 (75.002, -51.4258) -> (75.002, -41.1758) construction
  line L210 (80.8352, -43.8008) -> (85.8352, -43.8008) construction
  line L211 (85.8352, -43.8008) -> (85.8352, -48.8008) construction
  line L212 (85.8352, -48.8008) -> (80.8352, -48.8008) construction
  line L213 (80.8352, -48.8008) -> (80.8352, -43.8008) construction
  line L214 (83.3352, -41.1758) -> (83.3352, -51.4258) construction
  line L215 (75.002, -46.3008) -> (91.6685, -46.3008) construction
  line L216 (86.3352, -43.3008) -> (88.8352, -43.3008) construction
  line L217 (88.8352, -43.3008) -> (88.8352, -49.3008) construction
  line L218 (88.8352, -49.3008) -> (86.3352, -49.3008) construction
  line L219 (86.3352, -49.3008) -> (86.3352, -43.3008) construction
  line L220 (78.8352, -51.4258) -> (78.8352, -41.1758) construction
  line L221 (90.8352, -51.4258) -> (90.8352, -41.1758) construction
  line L222 (41.669, -41.1758) -> (58.3355, -41.1758) construction
  line L223 (58.3355, -41.1758) -> (58.3355, -51.4258) construction
  line L224 (58.3355, -51.4258) -> (41.669, -51.4258) construction
  line L225 (41.669, -51.4258) -> (41.669, -41.1758) construction
  line L226 (47.5022, -43.8008) -> (52.5022, -43.8008) construction
  line L227 (52.5022, -43.8008) -> (52.5022, -48.8008) construction
  line L228 (52.5022, -48.8008) -> (47.5022, -48.8008) construction
  line L229 (47.5022, -48.8008) -> (47.5022, -43.8008) construction
  line L230 (50.0022, -41.1758) -> (50.0022, -51.4258) construction
  line L231 (41.669, -46.3008) -> (58.3355, -46.3008) construction
  line L232 (53.0022, -43.3008) -> (55.5022, -43.3008) construction
  line L233 (55.5022, -43.3008) -> (55.5022, -49.3008) construction
  line L234 (55.5022, -49.3008) -> (53.0022, -49.3008) construction
  line L235 (53.0022, -49.3008) -> (53.0022, -43.3008) construction
  line L236 (45.5022, -51.4258) -> (45.5022, -41.1758) construction
  line L237 (57.5022, -51.4258) -> (57.5022, -41.1758) construction
  line L238 (91.6685, -41.1758) -> (108.335, -41.1758) construction
  line L239 (108.335, -41.1758) -> (108.335, -51.4258) construction
  line L240 (108.335, -51.4258) -> (91.6685, -51.4258) construction
  line L241 (91.6685, -51.4258) -> (91.6685, -41.1758) construction
  line L242 (97.5017, -43.8008) -> (102.5017, -43.8008) construction
  line L243 (102.5017, -43.8008) -> (102.5017, -48.8008) construction
  line L244 (102.5017, -48.8008) -> (97.5017, -48.8008) construction
  line L245 (97.5017, -48.8008) -> (97.5017, -43.8008) construction
  line L246 (100.0017, -41.1758) -> (100.0017, -51.4258) construction
  line L247 (91.6685, -46.3008) -> (108.335, -46.3008) construction
  line L248 (103.0017, -43.3008) -> (105.5017, -43.3008) construction
  line L249 (105.5017, -43.3008) -> (105.5017, -49.3008) construction
  line L250 (105.5017, -49.3008) -> (103.0017, -49.3008) construction
  line L251 (103.0017, -49.3008) -> (103.0017, -43.3008) construction
  line L252 (95.5017, -51.4258) -> (95.5017, -41.1758) construction
  line L253 (107.5017, -51.4258) -> (107.5017, -41.1758) construction
  line L254 (58.3355, -98.9103) -> (75.002, -98.9103) construction
  line L255 (75.002, -98.9103) -> (75.002, -109.1603) construction
  line L256 (75.002, -109.1603) -> (58.3355, -109.1603) construction
  line L257 (58.3355, -109.1603) -> (58.3355, -98.9103) construction
  line L258 (64.1687, -101.5353) -> (69.1687, -101.5353) construction
  line L259 (69.1687, -101.5353) -> (69.1687, -106.5353) construction
  line L260 (69.1687, -106.5353) -> (64.1687, -106.5353) construction
  line L261 (64.1687, -106.5353) -> (64.1687, -101.5353) construction
  line L262 (66.6687, -98.9103) -> (66.6687, -109.1603) construction
  line L263 (58.3355, -104.0353) -> (75.002, -104.0353) construction
  line L264 (69.6687, -101.0353) -> (72.1687, -101.0353) construction
  line L265 (72.1687, -101.0353) -> (72.1687, -107.0353) construction
  line L266 (72.1687, -107.0353) -> (69.6687, -107.0353) construction
  line L267 (69.6687, -107.0353) -> (69.6687, -101.0353) construction
  line L268 (62.1687, -109.1603) -> (62.1687, -98.9103) construction
  line L269 (74.1687, -109.1603) -> (74.1687, -98.9103) construction
  point P0 (73.3279, -41.0278)
  point P1 (116.6682, -17.4336)
  point P2 (116.6682, -17.4336)
  point P3 (100.0017, -17.4336)
  point P4 (100.0017, -17.4336)
  point P5 (83.3352, -75.1681)
  point P6 (100.0017, -46.3008)
  point P7 (66.6687, -104.0353)
  point P8 (83.3352, -17.4336)
  point P9 (66.6687, -17.4336)
  point P10 (33.3357, -17.4336)
  point P11 (16.6692, -17.4336)
  point P12 (100.0017, -46.3008)
  point P13 (83.3352, -46.3008)
  point P14 (66.6687, -46.3008)
  point P15 (50.0022, -46.3008)
  point P16 (33.3357, -46.3008)
  point P17 (50.0022, -75.1681)
  point P18 (66.6687, -75.1681)
  point P19 (83.3352, -75.1681)
  point P20 (66.6687, -104.0353)
  dimension "d56" = 16.6665
  dimension "d61" = 16.6665
  dimension "d62" = 28.8672
  measures "d56" distance from line of L9 L0.end
  measures "d61" distance from line of L0.start L3
  measures "d62" distance of L1.end L9.end